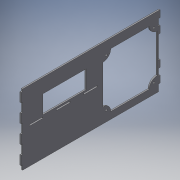
# Autodesk Inventor part: TrayPanelC
Saved by Autodesk Inventor 2017 (Build 210142000, 142)
## iProperties
Created: 2019-06-22
Part Number: TrayPanelC
Material: Generic
Document SubType Name: Modeling
Designer: DDeGo
Density: 1 g/cm^3
Appearance: Default
Author: DDeGo
Autodesk Inventor part; units mm, degrees
ref_plane "YZ Plane" through (0, 0, 0) normal (1, 0, 0) x (0, 1, 0)
ref_plane "XZ Plane" through (0, 0, 0) normal (0, 1, 0) x (-1, 0, 0)
ref_plane "XY Plane" through (0, 0, 0) normal (0, 0, 1) x (1, 0, 0)
sketch "Block1" plane through (0, 0, 0) normal (0, 0, 1) x (1, 0, 0)
  arc A0 (277.5, 135) -> (295, 117.5) centre (295, 135) ccw
  circle A1 centre (287.5, 127.5) radius 2
  line L0 (295, 117.5) -> (295, 32.5)
  line L1 (192.5, 135) -> (277.5, 135)
  circle A2 centre (182.5, 127.5) radius 2
  arc A3 (295, 32.5) -> (277.5, 15) centre (295, 15) ccw
  arc A4 (175, 117.5) -> (192.5, 135) centre (175, 135) ccw
  line L2 (175, 32.5) -> (175, 117.5)
  line L3 (277.5, 15) -> (192.5, 15)
  circle A5 centre (182.5, 22.5) radius 2
  arc A6 (192.5, 15) -> (175, 32.5) centre (175, 15) ccw
  circle A7 centre (287.5, 22.5) radius 2
  point P0 (235, 75)
sketch "Sketch1" plane through (0, 0, 0) normal (1, 0, 0) x (0, 1, 0)
  line L0 (300, 155) -> (300, 0)
  line L1 (0, 155) -> (300, 155)
  line L2 (0, 0) -> (0, 155)
  line L3 (0, 0) -> (300, 0)
  line L4 (0, 150.15) -> (-3, 150.15)
  line L5 (-3, 150.15) -> (-3, 130)
  line L6 (-3, 130) -> (0, 130)
  line L7 (0, 130) -> (0, 150.15)
  line L8 (0, 110.15) -> (-3, 110.15)
  line L9 (-3, 110.15) -> (-3, 90)
  line L10 (-3, 90) -> (0, 90)
  line L11 (0, 90) -> (0, 110.15)
  line L12 (0, 70.15) -> (-3, 70.15)
  line L13 (-3, 70.15) -> (-3, 50)
  line L14 (-3, 50) -> (0, 50)
  line L15 (0, 50) -> (0, 70.15)
  line L16 (0, 30.15) -> (-3, 30.15)
  line L17 (-3, 30.15) -> (-3, 10)
  line L18 (-3, 10) -> (0, 10)
  line L19 (0, 10) -> (0, 30.15)
  line L20 (300, 155) -> (303, 155)
  line L21 (303, 155) -> (303, 139.85)
  line L22 (303, 139.85) -> (300, 139.85)
  line L23 (300, 139.85) -> (300, 155)
  line L24 (300, 125) -> (303, 125)
  line L25 (303, 125) -> (303, 109.85)
  line L26 (303, 109.85) -> (300, 109.85)
  line L27 (300, 109.85) -> (300, 125)
  line L28 (300, 44.85) -> (303, 44.85)
  line L29 (303, 44.85) -> (303, 60)
  line L30 (303, 60) -> (300, 60)
  line L31 (300, 60) -> (300, 44.85)
  line L32 (300, 30) -> (303, 30)
  line L33 (303, 30) -> (303, 14.85)
  line L34 (303, 14.85) -> (300, 14.85)
  line L35 (300, 14.85) -> (300, 30)
  arc A0 (279.5, 135) -> (297, 117.5) centre (297, 135) ccw
  circle A1 centre (289.5, 127.5) radius 2
  line L36 (297, 117.5) -> (297, 32.5)
  line L37 (194.5, 135) -> (279.5, 135)
  circle A2 centre (184.5, 127.5) radius 2
  arc A3 (297, 32.5) -> (279.5, 15) centre (297, 15) ccw
  arc A4 (177, 117.5) -> (194.5, 135) centre (177, 135) ccw
  line L38 (177, 32.5) -> (177, 117.5)
  line L39 (279.5, 15) -> (194.5, 15)
  circle A5 centre (184.5, 22.5) radius 2
  arc A6 (194.5, 15) -> (177, 32.5) centre (177, 15) ccw
  circle A7 centre (289.5, 22.5) radius 2
  dimension "d2" = 300
  dimension "d3" = 155
  dimension "d4" = 15
  dimension "d5" = 3
  dimension "d6" = 20.15
  dimension "d7" = 3
  dimension "d8" = 40
  dimension "d9" = 40
  dimension "d10" = 40
  dimension "d11" = 10
  dimension "d26" = 15.15
  dimension "d27" = 3
  dimension "d28" = 30
  dimension "d30" = 65
  dimension "d31" = 30
  constraints: 73 end point, 16 parallel, 10 horizontal, 9 equal length, 9 point on line, 8 perpendicular, 2 collinear, 1 coincident, 1 vertical
  measures "d2" distance between parallel lines of L2 L0
  measures "d3" distance between parallel lines of L3 L1
  measures "d6" distance of L8.end L9.end
  measures "d7" distance of L4.start L4.end
  measures "d8" distance between parallel lines of L14 L18
  measures "d9" distance between parallel lines of L10 L14
  measures "d10" distance between parallel lines of L6 L10
  measures "d11" vertical distance of point (0, 0) L17.end
  measures "d26" distance of L20.end L21.end
  measures "d27" distance of L0.start L20.end
  measures "d28" distance of L20.end L24.end
  measures "d30" distance of L29.end L24.end
  measures "d31" distance of L32.end L29.end
extrude "Extrusion1" add sketch "Sketch1" along normal blind 2.75
sketch "Sketch2" plane through (0, 0, 0) normal (-1, 0, 0) x (0, 0, 1)
  line L0 (79.5, 165) -> (76.75, 165)
  line L1 (76.75, 165) -> (76.75, 135)
  line L2 (76.75, 135) -> (79.5, 135)
  line L3 (79.5, 135) -> (79.5, 165)
  line L4 (79.5, 105) -> (76.75, 105)
  line L5 (76.75, 105) -> (76.75, 75)
  line L6 (76.75, 75) -> (79.5, 75)
  line L7 (79.5, 75) -> (79.5, 105)
  line L8 (79.5, 45) -> (76.75, 45)
  line L9 (76.75, 45) -> (76.75, 15)
  line L10 (76.75, 15) -> (79.5, 15)
  line L11 (79.5, 15) -> (79.5, 45)
  line L12 (0, 0) -> (0, 300) projected
  line L13 (90, 0) -> (70.15, 0) projected
  point P0 (0, 303)
  dimension "d12" = 76.75
  dimension "d13" = 2.75
  dimension "d14" = 15
  dimension "d15" = 30
  dimension "d16" = 60
  dimension "d17" = 60
  constraints: 24 end point, 6 parallel, 3 equal length, 3 horizontal, 3 perpendicular, 2 point on line, 1 collinear
  measures "d12" distance between parallel lines of L12 L1
  measures "d13" distance of L1.end L2.end
  measures "d14" distance between parallel lines of L13 L10
  measures "d15" distance of L10.end L8.start
  measures "d16" distance of L9.end L5.end
  measures "d17" distance of L1.end L5.end
extrude "Extrusion2" cut sketch "Sketch2" against normal blind 10
sketch "Sketch3" plane through (2.75, 0, 0) normal (1, 0, 0) x (0, 0, -1)
  line L0 (-83.5, 140) -> (-123.5, 140)
  line L1 (-123.5, 140) -> (-123.5, 45)
  line L2 (-123.5, 45) -> (-83.5, 45)
  line L3 (-83.5, 45) -> (-83.5, 140)
  line L4 (-79.5, 75) -> (-79.5, 105) projected
  line L5 (-79.5, 105) -> (-76.75, 105) projected
  point P0 (0, 0)
  dimension "d20" = 4
  dimension "d21" = 35
  dimension "d22" = 60
  dimension "d23" = 40
  constraints: 8 end point, 2 parallel, 1 horizontal, 1 perpendicular
  measures "d20" distance between parallel lines of L3 L4
  measures "d21" distance between parallel lines of L5 L0
  measures "d22" distance between parallel lines of L2 L5
  measures "d23" distance of L0.start L0.end
extrude "Extrusion3" cut sketch "Sketch3" against normal blind 10
equation "\"d9\" = d8"
equation "\"d10\" = d8"
body "Solid1"
